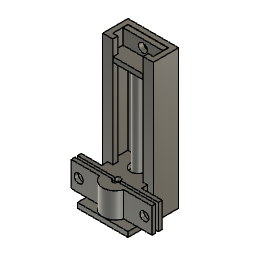
electrode_holder_spring (Autodesk Fusion 360 design; units mm, degrees)
Autodesk Fusion 360 part; units mm, degrees
note: some values were not read from the file. Chosen so that the rebuilt part matches the saved one: where a step ends. Set by a fixed rule: which sketch regions a step uses.
sketch "スケッチ1" plane through (0, 0, 0) normal (0, 0, 1) x (1, 0, 0)
  line L0 (10, 0) -> (-10, 0)
  line L1 (-10, 0) -> (-10, 10)
  line L2 (-10, 10) -> (10, 10)
  line L3 (10, 10) -> (10, 0)
  dimension "d1" = 20
  dimension "d2" = 10
  constraint horizontal L0
  constraint vertical L1
  constraint horizontal L2
  constraint vertical L3
  constraint midpoint origin L0
  measures "d1" distance of L0.start L0.end
  measures "d2" distance of L0.start L2.end
extrude "押し出し1" add sketch "スケッチ1" against normal blind 2 makes body 1
sketch "スケッチ3" plane through (0, 0, 0) normal (0, 0, 1) x (-1, 0, 0)
  line L0 (-10, -10) -> (10, -10)
  line L1 (10, -10) -> (10, 0)
  line L2 (10, 0) -> (-10, 0)
  line L3 (-10, 0) -> (-10, -10)
  line L4 (10, -10) -> (8, -10)
  line L5 (8, -10) -> (8, 0)
  line L6 (8, 0) -> (10, 0)
  line L7 (10, 0) -> (10, -10)
  line L8 (-10, -10) -> (10, -10)
  line L9 (10, -10) -> (10, -8)
  line L10 (10, -8) -> (-10, -8)
  line L11 (-10, -8) -> (-10, -10)
  line L12 (-10, 0) -> (-8, 0)
  line L13 (-8, 0) -> (-8, -10)
  line L14 (-8, -10) -> (-10, -10)
  line L15 (-10, -10) -> (-10, 0)
  dimension "d8" = 2
  dimension "d9" = 2
  dimension "d10" = 2
  constraint horizontal L4
  constraint vertical L5
  constraint horizontal L6
  constraint vertical L7
  constraint coincident L2 L5.end
  constraint coincident L0.end L1.start
  constraint horizontal L8
  constraint vertical L9
  constraint horizontal L10
  constraint vertical L11
  constraint coincident L7 L9.end
  constraint coincident L0.start L3.end
  constraint horizontal L12
  constraint vertical L13
  constraint horizontal L14
  constraint vertical L15
  constraint coincident L8 L13.end
  constraint coincident L2.end L3.start
  measures "d8" distance of L5 L7
  measures "d9" distance of L13 L15
  measures "d10" distance of L8 L10
extrude "押し出し3" add sketch "スケッチ3" along normal blind 53 contours L0 L3 L8 L10 L11 L13 L14 L15 | L0 L5 L8 L10 L13 | L2 L3 L10 L12 L13 L15 | L0 L1 L4 L5 L7 L8 L9 L10 | L1 L2 L5 L6 L7 L10 bodies 1
sketch "スケッチ2" plane through (0, 0, 0) normal (0, 0, 1) x (-1, 0, 0)
  line L0 (8, 0) -> (-8, 0)
  circle A0 centre (0, -4) radius 2
  line L1 (8, -8) -> (8, 0)
  line L2 (-8, 0) -> (-8, -8)
  line L3 (-8, -8) -> (8, -8)
  line L4 (0, -1.75) -> (0, -22.5)
  dimension "d5" = 4
  dimension "d14" = 4
  constraint coincident A0.centre L4
  measures "d5" diameter of A0
  measures "d14" distance of A0.centre L3
extrude "押し出し2" add sketch "スケッチ2" along normal blind 45 contours A0 L4 | A0 L4 bodies 1
sketch "スケッチ4" plane through (0, 0, 0) normal (0, 0, 1) x (-1, 0, 0)
  circle A0 centre (0, -4) radius 2
  line L0 (8, -8) -> (8, 0)
  line L1 (8, 0) -> (-8, 0)
  line L2 (-8, 0) -> (-8, -8)
  line L3 (-8, -8) -> (8, -8)
  line L4 (7.9, -7.9) -> (-7.9, -7.9)
  line L5 (-7.9, -7.9) -> (-7.9, 4)
  line L6 (-7.9, 4) -> (7.9, 4)
  line L7 (7.9, 4) -> (7.9, -7.9)
  circle A1 centre (0, -4) radius 2.125
  dimension "d15" = 4.25
  dimension "d16" = 0.1
  dimension "d17" = 0.1
  dimension "d18" = 0.1
  dimension "d19" = 4
  constraint horizontal L4
  constraint vertical L5
  constraint horizontal L6
  constraint vertical L7
  constraint concentric A0 A1
  measures "d15" diameter of A1
  measures "d16" distance of L3 L4
  measures "d17" distance of L2 L5
  measures "d18" distance of L0 L7
  measures "d19" distance of L1 L6
extrude "押し出し4" add sketch "スケッチ4" along normal blind 10 separate body contours L1 L4 L5 L7 | L1 L5 L6 L7 makes body 2
sketch "スケッチ5" plane through (0, 0, 0) normal (0, 0, -1) x (1, 0, 0)
  circle A0 centre (0, -4) radius 2.125
  line L0 (7.9, 4) -> (-7.9, 4)
  line L1 (-7.9, 4) -> (-7.9, -7.9)
  line L2 (-7.9, -7.9) -> (7.9, -7.9)
  line L3 (7.9, -7.9) -> (7.9, 4)
  arc A1 (-3, 4) -> (3, 4) centre (0, 4) ccw
  dimension "d22" = 6
  constraint midpoint L0 A1.centre
  constraint coincident L0 A1.end
  constraint coincident L0 A1.start
  measures "d22" diameter of A1
sketch "スケッチ17" plane through (0, 0, 10) normal (0, 0, 1) x (-1, 0, 0)
  circle A0 centre (0, -4) radius 2.125
  line L0 (7.9, 4) -> (-7.9, 4)
  line L1 (-7.9, 4) -> (-7.9, -7.9)
  line L2 (-7.9, -7.9) -> (7.9, -7.9)
  line L3 (7.9, -7.9) -> (7.9, 4)
  circle A1 centre (0, -4) radius 3
  dimension "d64" = 6
  constraint concentric A0 A1
  measures "d64" diameter of A1
extrude "押し出し16" cut sketch "スケッチ17" against normal blind 2 contours A1 bodies 2
extrude "押し出し5" cut sketch "スケッチ5" against normal blind 8.5 contours L0 A1 bodies 2
sketch "スケッチ6" plane through (0, 0, 10) normal (0, 0, 1) x (-1, 0, 0)
  line L0 (7.9, 4) -> (-7.9, 4)
  line L1 (-7.9, 4) -> (-7.9, -7.9)
  line L2 (-7.9, -7.9) -> (7.9, -7.9)
  line L3 (7.9, -7.9) -> (7.9, 4)
  arc A0 (-1.125, 4) -> (1.125, 4) centre (0, 4) ccw
  circle A1 centre (0, -4) radius 3
  dimension "d25" = 2.25
  constraint midpoint L0 A0.centre
  constraint coincident L0 A0.end
  constraint coincident L0 A0.start
  measures "d25" diameter of A0
extrude "押し出し6" cut sketch "スケッチ6" against normal up to surface (1.5 mm away) contours L0 A0 bodies 2
sketch "スケッチ7" plane through (0, -4, 0) normal (0, -1, 0) x (1, 0, 0)
  line L0 (1.125, 10) -> (1.125, 8.5)
  line L1 (1.125, 8.5) -> (3, 8.5)
  line L2 (3, 8.5) -> (3, 0)
  line L3 (3, 0) -> (7.9, 0)
  line L4 (7.9, 0) -> (7.9, 10)
  line L5 (7.9, 10) -> (1.125, 10)
  line L6 (7.9, 10) -> (16, 10)
  line L7 (16, 10) -> (16, 0)
  line L8 (16, 0) -> (7.9, 0)
  line L9 (7.9, 0) -> (7.9, 10)
  line L10 (10, -2) -> (10, 53)
  line L11 (-7.9, 10) -> (-16, 10)
  line L12 (-16, 10) -> (-16, 0)
  line L13 (-16, 0) -> (-7.9, 0)
  line L14 (-7.9, 0) -> (-7.9, 10)
  line L15 (-7.9, 0) -> (-7.9, 10)
  line L16 (-7.9, 10) -> (-1.125, 10)
  line L17 (-3, 0) -> (-7.9, 0)
  line L18 (-10, -2) -> (-10, 53)
  circle A0 centre (-13, 5) radius 1.75
  circle A1 centre (13, 5) radius 1.75
  line L19 (-13, 5) -> (13, 5) construction
  dimension "d28" = 6
  dimension "d29" = 6
  dimension "d30" = 3.5
  dimension "d31" = 3.5
  dimension "d32" = 3
  dimension "d33" = 3
  dimension "d34" = 5
  constraint horizontal L6
  constraint vertical L7
  constraint horizontal L8
  constraint vertical L9
  constraint coincident L4.end L5.start
  constraint collinear L3 L8
  constraint horizontal L11
  constraint vertical L12
  constraint horizontal L13
  constraint vertical L14
  constraint collinear L14 L15
  constraint collinear L11 L16
  constraint collinear L13 L17
  constraint coincident A0.centre L19.start
  constraint coincident A1.centre L19.end
  measures "d28" distance of L7 L10
  measures "d29" distance of L12 L18
  measures "d30" diameter of A0
  measures "d31" diameter of A1
  measures "d32" distance of L12 A0.centre
  measures "d33" distance of L7 A1.centre
  measures "d34" distance of L6 L19
extrude "押し出し7" add sketch "スケッチ7" against normal blind 1.5 contours L4 L6 L8 L9 L10 | L6 L7 L8 L10 | L11 L13 L14 L15 L18 | L11 L12 L13 L18 bodies 2
ref_plane "作業平面1" through (8.5625, -5, 5) normal (0, -1, 0) x (1, 0, 0)
sketch "スケッチ9" plane through (9.75, -5, 5) normal (0, -1, 0) x (1, 0, 0)
  circle A0 centre (-22.75, 0) radius 1.75
  line L0 (-10.875, 3.5) -> (-10.875, 5)
  line L1 (-10.875, 5) -> (-25.75, 5)
  line L2 (-25.75, 5) -> (-25.75, -5)
  line L3 (-25.75, -5) -> (-12.75, -5)
  line L4 (-12.75, -5) -> (-12.75, 3.5)
  line L5 (-12.75, 3.5) -> (-10.875, 3.5)
  line L6 (-8.625, 3.5) -> (-10.875, 3.5)
  line L7 (-8.625, 3.5) -> (-8.625, 5)
  line L8 (-10.875, 5) -> (-8.625, 5)
  line L9 (-10.875, 5) -> (-10.875, 3.5)
  circle A1 centre (3.25, 0) radius 1.75
  line L10 (-8.625, 5) -> (-8.625, 3.5)
  line L11 (-8.625, 3.5) -> (-6.75, 3.5)
  line L12 (-6.75, 3.5) -> (-6.75, -5)
  line L13 (-6.75, -5) -> (6.25, -5)
  line L14 (6.25, -5) -> (6.25, 5)
  line L15 (6.25, 5) -> (-8.625, 5)
  line L16 (-6.75, -5) -> (-12.75, -5)
  line L17 (-6.75, -5) -> (-6.75, 3.5)
  line L18 (-6.75, 3.5) -> (-12.75, 3.5)
  line L19 (-12.75, 3.5) -> (-12.75, -5)
extrude "押し出し8" add sketch "スケッチ9" along normal blind 1.5 separate body makes body 3
sketch "スケッチ10" plane through (0, 0, 10) normal (0, 0, 1) x (-1, 0, 0)
  line L0 (-16, 5) -> (16, 5)
  line L1 (16, 5) -> (16, 6.5)
  line L2 (16, 6.5) -> (-16, 6.5)
  line L3 (-16, 6.5) -> (-16, 5)
  arc A0 (5, 5) -> (-5, 5) centre (0, 5) ccw
  dimension "d40" = 10
  constraint midpoint L0 A0.centre
  constraint coincident L0 A0.end
  constraint coincident L0 A0.start
  measures "d40" diameter of A0
extrude "押し出し9" add sketch "スケッチ10" against normal blind 10 contours L0 L2 A0 | L2 A0 bodies 3
sketch "スケッチ11" plane through (0, 0, 0) normal (0, 0, -1) x (1, 0, 0)
  line L0 (-16, 5) -> (16, 5)
  line L1 (16, 5) -> (16, 6.5)
  line L2 (16, 6.5) -> (4.7697, 6.5)
  arc A0 (4.7697, 6.5) -> (-4.7697, 6.5) centre (0, 5) ccw
  line L3 (-4.7697, 6.5) -> (-16, 6.5)
  line L4 (-16, 6.5) -> (-16, 5)
  arc A1 (3, 5) -> (-3, 5) centre (0, 5) ccw
  dimension "d43" = 6
  constraint concentric A0 A1
  constraint coincident L0 A1.end
  constraint coincident L0 A1.start
  measures "d43" diameter of A1
extrude "押し出し10" cut sketch "スケッチ11" against normal blind 8.5 contours L0 A1 bodies 3
sketch "スケッチ12" plane through (0, 0, 10) normal (0, 0, 1) x (-1, 0, 0)
  line L0 (-16, 5) -> (16, 5)
  line L1 (16, 5) -> (16, 6.5)
  line L2 (16, 6.5) -> (4.7697, 6.5)
  arc A0 (4.7697, 6.5) -> (-4.7697, 6.5) centre (0, 5) ccw
  line L3 (-4.7697, 6.5) -> (-16, 6.5)
  line L4 (-16, 6.5) -> (-16, 5)
  arc A1 (1.125, 5) -> (-1.125, 5) centre (0, 5) ccw
  dimension "d46" = 2.25
  constraint concentric A0 A1
  constraint coincident L0 A1.end
  constraint coincident L0 A1.start
  measures "d46" diameter of A1
extrude "押し出し11" cut sketch "スケッチ12" along normal up to far side of body 3 contours L0 A1 bodies 3
sketch "スケッチ13" plane through (0, 0, 45) normal (0, 0, 1) x (-1, 0, 0)
  circle A0 centre (0, -4) radius 2
  line L0 (7.9, 0) -> (-7.9, 0)
  line L1 (-7.9, 2.5) -> (-7.9, -7.9)
  line L2 (7.9, -7.9) -> (7.9, 2.5)
  arc A1 (-1.125, 4) -> (1.125, 4) centre (0, 4) ccw
  line L3 (-1.125, 4) -> (-16, 4)
  line L4 (-16, 4) -> (-16, 2.5)
  line L5 (-16, 2.5) -> (-7.9, 2.5)
  line L6 (-7.9, 2.5) -> (-7.9, -7.9)
  line L7 (-7.9, -7.9) -> (7.9, -7.9)
  line L8 (7.9, -7.9) -> (7.9, 2.5)
  line L9 (7.9, 2.5) -> (16, 2.5)
  line L10 (16, 2.5) -> (16, 4)
  line L11 (16, 4) -> (1.125, 4)
  circle A2 centre (0, -4) radius 3
  constraint horizontal L0
  constraint coincident L0.end L1
  constraint coincident L0.start L2
  constraint midpoint origin L0
extrude "押し出し12" add sketch "スケッチ13" along normal blind 2 separate body contours A0 | L0 L1 L2 L6 L7 L8 | A2 makes body 4
sketch "スケッチ14" plane through (0, 0, 45) normal (0, 0, -1) x (1, 0, 0)
  line L0 (-7.9, 0) -> (-7.9, -7.9)
  line L1 (-7.9, -7.9) -> (7.9, -7.9)
  line L2 (7.9, -7.9) -> (7.9, 0)
  line L3 (7.9, 0) -> (-7.9, 0)
  circle A0 centre (0, -4) radius 3
  circle A1 centre (0, -4) radius 2
  dimension "d52" = 6
  constraint concentric A0 A1
  measures "d52" diameter of A0
extrude "押し出し13" cut sketch "スケッチ14" against normal blind 1 contours A0 | A1 bodies 4
sketch "スケッチ15" plane through (0, 7.9, 0) normal (0, 1, 0) x (-1, 0, 0)
  line L0 (-7.9, 45) -> (7.9, 45)
  line L1 (7.9, 45) -> (7.9, 47)
  line L2 (7.9, 47) -> (-7.9, 47)
  line L3 (-7.9, 47) -> (-7.9, 45)
  line L4 (-7.9, 47) -> (7.9, 47)
  line L5 (7.9, 47) -> (7.9, 53)
  line L6 (7.9, 53) -> (-7.9, 53)
  line L7 (-7.9, 53) -> (-7.9, 47)
  dimension "d55" = 6
  constraint horizontal L4
  constraint vertical L5
  constraint horizontal L6
  constraint vertical L7
  constraint coincident L2.end L3.start
  constraint collinear L1 L5
  measures "d55" distance of L2.end L6.end
extrude "押し出し14" add sketch "スケッチ15" against normal blind 2 contours L2 L4 L5 L6 L7 bodies 4
sketch "スケッチ16" plane through (0, 5.9, 0) normal (0, -1, 0) x (1, 0, 0)
  line L0 (7.9, 47) -> (7.9, 53)
  line L1 (7.9, 53) -> (-7.9, 53)
  line L2 (-7.9, 53) -> (-7.9, 47)
  line L3 (-7.9, 47) -> (7.9, 47)
  circle A0 centre (0, 50) radius 1.75
  dimension "d61" = 3.5
  dimension "d67" = 3
  measures "d61" diameter of A0
  measures "d67" distance of L1 A0.centre
extrude "押し出し15" cut sketch "スケッチ16" against normal up to surface (4.1 mm away) contours A0 bodies 1 4
sketch "スケッチ23" plane through (0, 0, 0) normal (0, 0, 1) x (-1, 0, 0)
  circle A0 centre (0, -4) radius 2
  line L0 (8, -8) -> (8, 0)
  line L1 (8, 0) -> (-8, 0)
  line L2 (-8, 0) -> (-8, -8)
  line L3 (-8, -8) -> (8, -8)
  line L4 (-8, 0) -> (-6, 0)
  line L5 (-6, 0) -> (-6, -2)
  line L6 (-6, -2) -> (-8, -2)
  line L7 (-8, -2) -> (-8, 0)
  line L8 (8, 0) -> (6, 0)
  line L9 (6, 0) -> (6, -2)
  line L10 (6, -2) -> (8, -2)
  line L11 (8, -2) -> (8, 0)
  dimension "d72" = 2
  dimension "d73" = 2
  dimension "d74" = 2
  dimension "d75" = 2
  constraint horizontal L4
  constraint vertical L5
  constraint horizontal L6
  constraint vertical L7
  constraint coincident L1.end L2.start
  constraint horizontal L8
  constraint vertical L9
  constraint horizontal L10
  constraint vertical L11
  constraint coincident L0.end L1.start
  measures "d72" distance of L1.end L4.end
  measures "d73" distance of L4.end L5.end
  measures "d74" distance of L8.end L9.end
  measures "d75" distance of L9.end L10.end
extrude "押し出し18" add sketch "スケッチ23" along normal up to surface (53 mm away) contours L0 L1 L8 L9 L10 L11 | L1 L2 L4 L5 L6 L7 bodies 1
sketch "スケッチ24" plane through (0, 0, 10) normal (0, 0, 1) x (-1, 0, 0)
  arc A0 (-1.125, 4) -> (1.125, 4) centre (0, 4) ccw
  line L0 (-1.125, 4) -> (-16, 4)
  line L1 (-16, 4) -> (-16, 2.5)
  line L2 (-16, 2.5) -> (-7.9, 2.5)
  line L3 (-7.9, 2.5) -> (-7.9, -7.9)
  line L4 (-7.9, -7.9) -> (7.9, -7.9)
  line L5 (7.9, -7.9) -> (7.9, 2.5)
  line L6 (7.9, 2.5) -> (16, 2.5)
  line L7 (16, 2.5) -> (16, 4)
  line L8 (16, 4) -> (1.125, 4)
  circle A1 centre (0, -4) radius 3
  line L9 (-7.9, -2.1) -> (-5.9, -2.1)
  line L10 (-5.9, -2.1) -> (-5.9, 0.1)
  line L11 (-5.9, 0.1) -> (-7.9, 0.1)
  line L12 (-7.9, 0.1) -> (-7.9, -2.1)
  line L13 (-10, -10) -> (10, -10)
  line L14 (10, -10) -> (10, 0)
  line L15 (10, 0) -> (6, 0)
  line L16 (6, 0) -> (6, -2)
  line L17 (6, -2) -> (8, -2)
  line L18 (8, -2) -> (8, -8)
  line L19 (8, -8) -> (-8, -8)
  line L20 (-8, -8) -> (-8, -2)
  line L21 (-8, -2) -> (-6, -2)
  line L22 (-6, -2) -> (-6, 0)
  line L23 (-6, 0) -> (-10, 0)
  line L24 (-10, 0) -> (-10, -10)
  line L25 (7.9, -2.1) -> (5.9, -2.1)
  line L26 (5.9, -2.1) -> (5.9, 0.1)
  line L27 (5.9, 0.1) -> (7.9, 0.1)
  line L28 (7.9, 0.1) -> (7.9, -2.1)
  dimension "d78" = 0.1
  dimension "d79" = 0.1
  dimension "d80" = 0.1
  dimension "d81" = 0.1
  dimension "d82" = 0.1
  dimension "d83" = 0.1
  constraint horizontal L9
  constraint vertical L10
  constraint horizontal L11
  constraint vertical L12
  constraint coincident L3 L9.start
  constraint horizontal L25
  constraint vertical L26
  constraint horizontal L27
  constraint vertical L28
  constraint coincident L5 L25.start
  measures "d78" distance of L9 L21
  measures "d79" distance of L10 L22
  measures "d80" distance of L11 L23
  measures "d81" distance of L17 L25
  measures "d82" distance of L16 L26
  measures "d83" distance of L15 L27
extrude "押し出し19" cut sketch "スケッチ24" against normal up to surface (10 mm away) contours L3 L9 L10 L11 L12 L21 L22 L23 | L5 L15 L16 L17 L25 L26 L27 L28 | L3 L12 L21 L22 L23 | L5 L15 L16 L17 L28 bodies 2
sketch "スケッチ25" plane through (0, 0, 47) normal (0, 0, 1) x (-1, 0, 0)
  line L0 (-7.9, -5.9) -> (7.9, -5.9)
  line L1 (7.9, -5.9) -> (7.9, 0)
  line L2 (7.9, 0) -> (-7.9, 0)
  line L3 (-7.9, 0) -> (-7.9, -5.9)
  line L4 (7.9, -2.1) -> (5.9, -2.1)
  line L5 (5.9, -2.1) -> (5.9, 0)
  line L6 (5.9, 0) -> (7.9, 0)
  line L7 (7.9, 0) -> (7.9, -2.1)
  line L8 (-10, -10) -> (10, -10)
  line L9 (10, -10) -> (10, 0)
  line L10 (10, 0) -> (6, 0)
  line L11 (6, 0) -> (6, -2)
  line L12 (6, -2) -> (8, -2)
  line L13 (8, -2) -> (8, -8)
  line L14 (8, -8) -> (-8, -8)
  line L15 (-8, -8) -> (-8, -2)
  line L16 (-8, -2) -> (-6, -2)
  line L17 (-6, -2) -> (-6, 0)
  line L18 (-6, 0) -> (-10, 0)
  line L19 (-10, 0) -> (-10, -10)
  line L20 (-7.9, -2.1) -> (-5.9, -2.1)
  line L21 (-5.9, -2.1) -> (-5.9, 0)
  line L22 (-5.9, 0) -> (-7.9, 0)
  line L23 (-7.9, 0) -> (-7.9, -2.1)
  dimension "d86" = 0.1
  dimension "d87" = 0.1
  dimension "d88" = 0.1
  dimension "d89" = 0.1
  constraint horizontal L4
  constraint vertical L5
  constraint horizontal L6
  constraint vertical L7
  constraint coincident L2 L5.end
  constraint coincident L1 L4.start
  constraint horizontal L20
  constraint vertical L21
  constraint horizontal L22
  constraint vertical L23
  constraint coincident L2 L21.end
  constraint coincident L3 L20.start
  measures "d86" distance of L4 L12
  measures "d87" distance of L5 L11
  measures "d88" distance of L16 L20
  measures "d89" distance of L17 L21
extrude "押し出し20" cut sketch "スケッチ25" against normal up to surface (2 mm away) contours L2 L3 L16 L17 L20 L21 L22 L23 | L1 L2 L4 L5 L6 L7 L11 L12 | L2 L3 L16 L17 L18 L22 L23 | L1 L2 L6 L7 L10 L11 L12 bodies 4
sketch "スケッチ26" plane through (0, 0, -2) normal (0, 0, -1) x (1, 0, 0)
  line L0 (-10, -10) -> (10, -10)
  line L1 (10, -10) -> (10, 0)
  line L2 (10, 0) -> (-10, 0)
  line L3 (-10, 0) -> (-10, -10)
  line L4 (10, 0) -> (-10, 0)
  line L5 (-10, 0) -> (-10, 10)
  line L6 (-10, 10) -> (10, 10)
  line L7 (10, 10) -> (10, 0)
  arc A0 (3, 5) -> (-3, 5) centre (0, 5) ccw
  line L8 (3, 5) -> (16, 5)
  line L9 (16, 5) -> (16, 6.5)
  line L10 (16, 6.5) -> (4.7697, 6.5)
  arc A1 (4.7697, 6.5) -> (-4.7697, 6.5) centre (0, 5) ccw
  line L11 (-4.7697, 6.5) -> (-16, 6.5)
  line L12 (-16, 6.5) -> (-16, 5)
  line L13 (-16, 5) -> (-3, 5)
  circle A2 centre (0, -4) radius 2.125
  line L14 (-7.9, 0.1) -> (-5.9, 0.1)
  line L15 (-5.9, 0.1) -> (-5.9, -2.1)
  line L16 (-5.9, -2.1) -> (-7.9, -2.1)
  line L17 (-7.9, -2.1) -> (-7.9, -7.9)
  line L18 (-7.9, -7.9) -> (7.9, -7.9)
  line L19 (7.9, -7.9) -> (7.9, -2.1)
  line L20 (7.9, -2.1) -> (5.9, -2.1)
  line L21 (5.9, -2.1) -> (5.9, 0.1)
  line L22 (5.9, 0.1) -> (7.9, 0.1)
  line L23 (7.9, 0.1) -> (7.9, 2.5)
  line L24 (7.9, 2.5) -> (16, 2.5)
  line L25 (16, 2.5) -> (16, 4)
  line L26 (16, 4) -> (3, 4)
  arc A3 (-3, 4) -> (3, 4) centre (0, 4) ccw
  line L27 (-3, 4) -> (-16, 4)
  line L28 (-16, 4) -> (-16, 2.5)
  line L29 (-16, 2.5) -> (-7.9, 2.5)
  line L30 (-7.9, 2.5) -> (-7.9, 0.1)
  line L31 (-3, 5) -> (3, 4) construction
  line L32 (3, 5) -> (-3, 4) construction
  circle A4 centre (0, 4.5) radius 3.15
  dimension "d92" = 6.3
  constraint horizontal L4
  constraint vertical L5
  constraint horizontal L6
  constraint vertical L7
  constraint coincident L1.end L2.start
  constraint tangent L6 A1
  constraint collinear L3 L5
  constraint coincident A0.end L13.end
  constraint coincident L26.end A3.end
  constraint coincident A0.start L8.start
  constraint coincident A3.start L27.start
  constraint midpoint L32 A4.centre
  measures "d92" diameter of A4
extrude "押し出し21" add sketch "スケッチ26" against normal up to surface (2 mm away) contours L2 L4 L5 L14 L15 L29 L30 | L2 L4 L7 L21 L22 L23 L24 | L2 L4 L5 L7 L14 L15 L21 L22 L23 L24 L26 A3 L27 L29 L30 A4 | L5 L13 L27 A4 | L7 L8 L26 A4 | L5 L7 A0 L8 L10 A1 L11 L13 A4 | L5 L6 A1 L11 | A3 A4 | L6 L7 L10 A1 | A0 A4 bodies 1
